Motor_v4 (Autodesk Fusion 360 design; units mm, degrees)
Autodesk Fusion 360 part; units mm, degrees
sketch "Esquisse1" plane through (0, 0, 0) normal (0, 0, 1) x (1, 0, 0) in component "Motor"
  line L0 (0, 0) -> (0, 16.99)
  line L1 (0, 16.99) -> (15.3, 16.99)
  line L2 (15.3, 16.99) -> (15.3, 0)
  line L3 (46.1, 17) -> (46.1, 0)
  line L4 (46.1, 0) -> (67.6, 0) construction
  line L5 (67.6, 0) -> (67.6, 18.5)
  line L6 (67.6, 18.5) -> (46.1, 18.5)
  line L7 (46.1, 18.5) -> (46.1, 17)
  line L8 (0, 0) -> (67.6, 0)
  line L9 (15.3, 16.99) -> (15.3, 17)
  line L10 (15.3, 17) -> (46.1, 17)
  dimension "d2" = 16.99
  dimension "d7" = 15.3
  dimension "d8" = 30.8
  dimension "d10" = 21.5
  dimension "d11" = 18.5
  dimension "d12" = 21.5
  dimension "d13" = 0.01
  constraint coincident L0.start L8.start
  constraint perpendicular L0 L1
  constraint perpendicular L3 L4
  constraint perpendicular L4 L5
  constraint perpendicular L5 L6
  constraint perpendicular L5 L8
  constraint horizontal L8
  constraint horizontal L1
  constraint vertical L9
  constraint horizontal L10
  constraint vertical L2
  measures "d2" distance of L0.start L0.end
  measures "d7" distance of L0.end L1.end
  measures "d8" distance of L1.end L3.start
  measures "d10" distance of L3.end L4.end
  measures "d11" distance of L4.end L5.end
  measures "d12" distance of L5.end L6.end
  measures "d13" distance of L1.end L9.end
revolve "Révolution1" add sketch "Esquisse1" angle 360 about axis through (0, 0, 0) along (1, 0, 0) makes body 1 in component "Motor"
sketch "Esquisse2" plane through (67.6, 0, 0) normal (1, 0, 0) x (0, 1, 0) in component "Motor"
  circle A0 centre (0, 0) radius 18.5
  line L0 (0, 0) -> (18.5, 0) construction
  line L1 (0, 0) -> (-15.5, 0) construction
  circle A1 centre (-15.5, 0) radius 1.5
  circle A2 centre (0, 0) radius 15.5 construction
  line L2 (-15.5, 0) -> (-7.75, -13.4234) construction
  circle A3 centre (-7.75, -13.4234) radius 1.5
  circle A4 centre (-7.75, 13.4234) radius 1.5
  line L3 (0, 0) -> (0, -18.5) construction
  circle A5 centre (7.75, 13.4234) radius 1.5
  circle A6 centre (15.5, 0) radius 1.5
  circle A7 centre (7.75, -13.4234) radius 1.5
  line L4 (0, 0) -> (0, -7) construction
  circle A8 centre (0, -7) radius 6
  circle A9 centre (0, -7) radius 3
  dimension "d14" = 15.5
  dimension "d15" = 3
  dimension "d16" = 15.5
  dimension "d17" = 3
  dimension "d18" = 7
  dimension "d19" = 12
  dimension "d20" = 6
  dimension "d27" = 3
  dimension "d28" = 3
  dimension "d29" = 3
  dimension "d30" = 3
  constraint coincident A0.centre L0.start
  constraint coincident A0 L0.end
  constraint horizontal L0
  constraint parallel L0 L1
  constraint coincident L1.end A1.centre
  constraint concentric A0 A2
  constraint coincident L1.end A2
  constraint coincident A2 L2.end
  constraint coincident L2.end A3.centre
  constraint symmetric L1 A3 A4
  constraint coincident A0 L3.end
  constraint perpendicular L0 L3
  constraint symmetric A1 L3 A6
  constraint symmetric A3 L3 A7
  constraint symmetric A4 L3 A5
  constraint perpendicular L0 L4
  constraint coincident L4.end A8.centre
  constraint concentric A8 A9
  measures "d14" distance of A0.centre L1.end
  measures "d15" diameter of A1
  measures "d16" distance of L1.end L2.end
  measures "d17" diameter of A3
  measures "d18" distance of A0.centre L4.end
  measures "d19" diameter of A8
  measures "d20" diameter of A9
  measures "d27" diameter of A7
  measures "d28" diameter of A6
  measures "d29" diameter of A5
  measures "d30" diameter of A4
extrude "Extrusion3" cut sketch "Esquisse2" against normal blind 10 contours A1 | A3 | A4 | A5 | A6 | A7 bodies 1 in component "Motor"
extrude "Extrusion1" add sketch "Esquisse2" along normal blind 6 contours A8 bodies 1 in component "Motor"
extrude "Extrusion2" add 1 faces at (67.6, -1.8565, -7.7286) along direction (1, 0, 0) blind 22 on bodies 1 bodies 1 in component "Motor"
copy_body "CutPasteBodies1" bodies 1 removing the originals makes body 2 in component "Motor"
component "Motor" placed x (1, 0, 0) y (0, 1, 0) z (0, 0, 1) at (0, 0, 0)
equation "d2 = ( ( 34 / 2 ) * 1 ) * 1 mm - 0.01 mm"
equation "d11 = ( 37 / 2 ) * 1 mm"
equation "d14 = ( 31 / 2 ) * 1 mm"
equation "d17 = d15"
